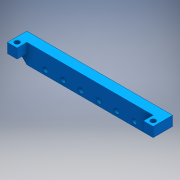
# Autodesk Inventor part: frameBottomRight
Saved by Autodesk Inventor 2016 (Build 200138000, 138)
## iProperties
Created: 2016-05-25
Part Number: frameBottomRight
Material: ABS Plastic
Document SubType Name: Modeling
Designer: Henrik Samuelsson
Density: 1.06 g/cm^3
Appearance: Smooth - White
Author: Henrik Samuelsson
Autodesk Inventor part; units mm, degrees
ref_plane "YZ Plane" through (0, 0, 0) normal (1, 0, 0) x (0, 1, 0)
ref_plane "XZ Plane" through (0, 0, 0) normal (0, 1, 0) x (-1, 0, 0)
ref_plane "XY Plane" through (0, 0, 0) normal (0, 0, 1) x (1, 0, 0)
sketch "Sketch5" plane through (0, 0, 0) normal (0, 1, 0) x (-1, 0, 0)
  line L0 (0, 0) -> (180, 0)
  line L1 (180, 0) -> (180, -12)
  line L2 (0, -12) -> (0, 0)
  line L3 (168, -24) -> (12, -24)
  line L4 (0, -12) -> (12, -24)
  line L5 (180, -12) -> (168, -24)
  circle A0 centre (101, -18) radius 3
  circle A1 centre (79, -18) radius 3
  circle A2 centre (57, -18) radius 3
  circle A3 centre (123, -18) radius 3
  circle A4 centre (145, -18) radius 3
  circle A5 centre (35, -18) radius 3
  dimension "d57" = 6
  dimension "d58" = 79
  dimension "d59" = 180
  dimension "d60" = 12
  dimension "d61" = 12
  dimension "d62" = 12
  dimension "d63" = 12
  dimension "d64" = 12
  dimension "d65" = 156
  dimension "d66" = 6
  dimension "d67" = 6
  dimension "d68" = 6
  dimension "d69" = 6
  dimension "d70" = 6
  dimension "d71" = 6
  dimension "d72" = 6
  dimension "d73" = 6
  dimension "d74" = 6
  dimension "d75" = 22
  dimension "d76" = 22
  dimension "d77" = 22
  dimension "d78" = 22
  dimension "d95" = 6
  dimension "d96" = 0
  dimension "d97" = 22
  constraints: 12 end point, 6 centre point, 1 horizontal, 1 parallel, 1 perpendicular
  measures "d57" diameter of A0
  measures "d58" distance from line of L1 A0.centre
  measures "d59" distance of L0.end L0.start
  measures "d60" distance of L0.start L2.start
  measures "d61" horizontal distance of L2.start L3.end
  measures "d62" horizontal distance of L1.end L3.start
  measures "d63" horizontal distance of L1.end L3.start
  measures "d64" horizontal distance of L3.end L2.start
  measures "d65" distance of L3.start L3.end
  measures "d66" distance from line of L3 A0.centre
  measures "d67" diameter of A1
  measures "d68" diameter of A2
  measures "d69" diameter of A3
  measures "d70" diameter of A4
  measures "d71" distance from line of L3 A2.centre
  measures "d72" distance from line of L3 A1.centre
  measures "d73" distance from line of L3 A3.centre
  measures "d74" distance from line of L3 A4.centre
  measures "d75" distance of A0.centre A1.centre
  measures "d76" distance of A1.centre A2.centre
  measures "d77" distance of A3.centre A0.centre
  measures "d78" distance of A4.centre A3.centre
  measures "d95" diameter of A5
  measures "d96" vertical distance of A2.centre A5.centre
  measures "d97" distance of A2.centre A5.centre
extrude "Extrusion7" add sketch "Sketch5" along normal blind 12
sketch "Sketch8" plane through (0, 0, 0) normal (0, -1, 0) x (1, 0, 0)
  line L0 (0, 0) -> (0, -12) projected
  line L1 (0, 0) -> (-12, 0)
  line L2 (-12, 0) -> (-12, -12)
  line L3 (-12, -12) -> (0, -12)
  line L4 (0, -12) -> (0, 0)
  line L5 (-180, -12) -> (-180, 0) projected
  line L6 (-180, 0) -> (-168, 0)
  line L7 (-168, 0) -> (-168, -12)
  line L8 (-168, -12) -> (-180, -12)
  line L9 (-180, -12) -> (-180, 0)
  dimension "d100" = 12
  dimension "d101" = 12
  dimension "d102" = 12
  dimension "d103" = 12
  constraints: 16 end point, 4 parallel, 2 horizontal, 2 perpendicular
  measures "d100" distance of L3.end L2.end
  measures "d101" distance of L2.end L1.end
  measures "d102" distance of L7.end L8.end
  measures "d103" distance of L6.end L7.end
extrude "Extrusion8" add sketch "Sketch8" along normal blind 12
sketch "Sketch9" plane through (-180, 12, 0) normal (0, 0, 1) x (1, 0, 0)
  circle A0 centre (174, -18) radius 3
  line L0 (180, -24) -> (168, -24) projected
  line L1 (180, -24) -> (180, 0) projected
  circle A1 centre (6, -18) radius 3
  line L2 (0, 0) -> (0, -24) projected
  line L3 (12, -24) -> (0, -24) projected
  point P0 (180, -12)
  dimension "d106" = 6
  dimension "d107" = 6
  dimension "d108" = 6
  dimension "d109" = 6
  dimension "d110" = 6
  dimension "d111" = 6
  constraints: 2 centre point
  measures "d106" diameter of A0
  measures "d107" distance from line of L0 A0.centre
  measures "d108" distance from line of A0.centre L1
  measures "d109" diameter of A1
  measures "d110" distance from line of L2 A1.centre
  measures "d111" distance from line of A1.centre L3
extrude "Extrusion9" cut sketch "Sketch9" against normal up to next
body "Solid2"
